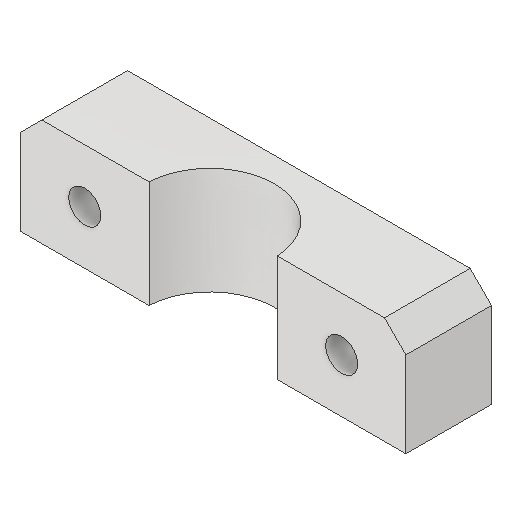
# Autodesk Inventor part: 3DP_PLA_X_axis_carriage_laser_mount_clamp
Saved by Autodesk Inventor 2025 (Build 290162010, 162A)
## iProperties
Created: 2018-08-01
Part Number: 3DP_PLA_X_axis_carriage_laser_mount_clamp
Material: ABS Plastic
Document SubType Name: Modeling
Designer: Andrzej
Density: 1.06 g/cm^3
Appearance: Smooth - White
Author: Andrzej
Autodesk Inventor part; units mm, degrees
ref_plane "YZ Plane" through (0, 0, 0) normal (1, 0, 0) x (0, 1, 0)
ref_plane "XZ Plane" through (0, 0, 0) normal (0, 1, 0) x (-1, 0, 0)
ref_plane "XY Plane" through (0, 0, 0) normal (0, 0, 1) x (1, 0, 0)
sketch "Sketch1" plane through (0, 0, 0) normal (0, 0, 1) x (1, 0, 0)
  line L0 (-8.7244, 5.8803) -> (27.2756, 5.8803)
  line L1 (27.2756, 5.8803) -> (27.2756, -4.1197)
  line L2 (27.2756, -4.1197) -> (-8.7244, -4.1197)
  line L3 (-8.7244, -4.1197) -> (-8.7244, 5.8803)
  point P0 (0, 0)
  point P1 (-2.7244, 0.8803)
  point P2 (21.2756, 0.8803)
  dimension "d0" = 36
  dimension "d1" = 24
  dimension "d2" = 6
  dimension "d3" = 10
  dimension "d4" = 5
  constraints: 8 end point, 2 parallel, 1 horizontal, 1 horizontal alignment, 1 perpendicular
  measures "d0" distance of L1.end L2.end
  measures "d1" distance of point (21.276, 0.88) point (-2.724, 0.88)
  measures "d2" distance from line of L3 point (-2.724, 0.88)
  measures "d3" distance between parallel lines of L2 L0
  measures "d4" distance from line of L0 point (-2.724, 0.88)
extrude "Extrusion1" add sketch "Sketch1" along normal blind 8
hole "Hole1" at (-2.7244, 0.8803, 0) at (21.2756, 0.8803, 0) direction (0, 0, 1) diameter 3 end through all
sketch "Sketch2" plane through (-8.7244, 5.8803, 0) normal (0, 1, 0) x (1, 0, 0)
  line L0 (0, 0) -> (36, 0) projected
  line L1 (0, 0) -> (0, -8) projected
  line L2 (36, -8) -> (0, -8) projected
  line L3 (36, 0) -> (36, -8) projected
  line L4 (0, -8) -> (36, -8) projected
  circle A0 centre (18, -8.3) radius 6
  point P0 (8.7244, 0)
  dimension "d15" = 36
  dimension "d22" = 12
  dimension "d23" = 18
  dimension "d24" = 0.3
  constraints: 1 centre point
  measures "d15" distance between parallel lines of L3 L1
  measures "d22" diameter of A0
  measures "d23" distance from line of L1 A0.centre
  measures "d24" distance from line of L2 A0.centre
extrude "Extrusion2" cut sketch "Sketch2" against normal through all contours A0 L2 | L2 A0
chamfer "Chamfer1" distance 2 angle 45 2 edges at (27.2756, 5.8803, 4) (-8.7244, 5.8803, 4)
equation "\"d2\" = -0.5 * d1 + 0.5 * d0"
equation "\"d23\" = 0.5 * d15"
body "Solid1"
